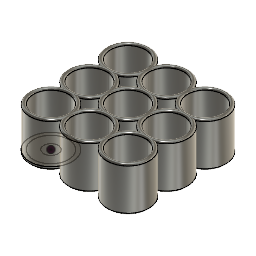
batteryholderAA (Autodesk Fusion 360 design; units mm, degrees)
Autodesk Fusion 360 part; units mm, degrees
sketch "Sketch2" plane through (0, 0, 0) normal (0, 0, 1) x (1, 0, 0)
  circle A0 centre (0, 0) radius 7.25
  circle A1 centre (0, 0) radius 8.75
  circle A2 centre (0, 0) radius 3
  dimension "d1" = 14.5
  dimension "d2" = 1.5
  dimension "d16" = 6
  measures "d1" diameter of A0
  measures "d16" diameter of A2
extrude "Extrude1" add sketch "Sketch2" along normal blind 1.5 contours A0 | A1 makes body 1
sketch "Sketch3" plane through (0, 0, 1.5) normal (0, 0, 1) x (-1, 0, 0)
  circle A0 centre (0, 0) radius 3
  circle A1 centre (0, 0) radius 8.75
extrude "Extrude2" cut sketch "Sketch3" against normal blind 1.5 bodies 1
extrude "Extrude3" add sketch "Sketch2" against normal blind 1.5 contours A0 | A1 bodies 1
extrude "Extrude4" add sketch "Sketch2" along normal blind 18.5 contours A1 bodies 1
extrude "Extrude5" cut 1 faces at (8.1904, -0.7949, 18.5) along direction (0, 0, -1) blind 11.5 on bodies 1 bodies 1
extrude "Extrude6" add 1 faces at (8.1904, -0.7949, 7) along direction (0, 0, 1) blind 10 on bodies 1 bodies 1
fillet "Fillet5" radius 0.75 1 edges at (-8.1579, -3.1641, 17) on bodies 1
fillet "Fillet6" radius 0.75 1 edges at (-6.7594, 2.6217, 17) on bodies 1
fillet "Fillet1" [no effect]
fillet "Fillet4" [no effect]
fillet "Fillet2" [no effect]
fillet "Fillet3" radius 0.75 1 edges at (-8.1579, 3.1641, -1.5) on bodies 1
copy_body "CopyPasteBodies5" bodies 1 makes body 2
move_body "Move5" bodies 2 to x (1, 0, 0) y (0, 1, 0) z (0, 0, 1) at (16.5, 0, 0)
copy_body "CopyPasteBodies6" bodies 2 makes body 3
move_body "Move6" bodies 3 to x (1, 0, 0) y (0, 1, 0) z (0, 0, 1) at (16.5, 0, 0)
copy_body "CopyPasteBodies7" bodies 1 2 3 makes body 4 makes body 5 makes body 6
move_body "Move7" bodies 4 5 6 to x (1, 0, 0) y (0, 1, 0) z (0, 0, 1) at (0, 16.5, 0)
copy_body "CopyPasteBodies8" bodies 1 2 3 makes body 7 makes body 8 makes body 9
move_body "Move8" bodies 7 8 9 to x (1, 0, 0) y (0, 1, 0) z (0, 0, 1) at (0, 33, 0)
move_body "Move9" bodies 8 3 9 2 5 6 to x (1, 0, 0) y (0, 1, 0) z (0, 0, 1) at (-0.5, 0, 0)
move_body "Move10" bodies 9 3 6 to x (1, 0, 0) y (0, 1, 0) z (0, 0, 1) at (-0.5, 0, 0)
move_body "Move11" bodies 8 7 9 6 4 5 to x (1, 0, 0) y (0, 1, 0) z (0, 0, 1) at (0, -0.5, 0)
move_body "Move12" bodies 8 7 9 to x (1, 0, 0) y (0, 1, 0) z (0, 0, 1) at (0, -0.5, 0)
